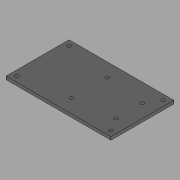
# Autodesk Inventor part: rfid_cover
Saved by Autodesk Inventor 2019 (Build 230136000, 136)
## iProperties
Part Number: rfid_cover
Material: Generic
Document SubType Name: Modeling
Designer: Javi
Appearance: Default
Author: Javi
Autodesk Inventor part; units mm, degrees
ref_plane "YZ Plane" through (0, 0, 0) normal (1, 0, 0) x (0, 1, 0)
ref_plane "XZ Plane" through (0, 0, 0) normal (0, 1, 0) x (-1, 0, 0)
ref_plane "XY Plane" through (0, 0, 0) normal (0, 0, 1) x (1, 0, 0)
sketch "Sketch1" plane through (0, 0, 0) normal (0, 1, 0) x (-1, 0, 0)
  line L0 (0, -60) -> (-100, -60)
  line L1 (-100, -60) -> (-100, 0)
  line L2 (-100, 0) -> (0, 0)
  line L3 (0, 0) -> (0, -60)
  dimension "d0" = 100
  dimension "d1" = 60
  constraints: 8 end point, 2 parallel, 1 coincident, 1 horizontal, 1 perpendicular
  measures "d0" distance of L0.start L0.end
  measures "d1" distance of L0.end L1.end
extrude "Extrusion1" add sketch "Sketch1" along normal blind 3
sketch "Sketch2" plane through (0, 3, 0) normal (0, 1, 0) x (1, 0, 0)
  circle A0 centre (5, 55) radius 1.75
  line L0 (100, 60) -> (0, 60) projected
  line L1 (0, 60) -> (0, 0) projected
  circle A1 centre (95, 55) radius 1.75
  circle A2 centre (5, 5) radius 1.75
  circle A3 centre (95, 5) radius 1.75
  circle A4 centre (87.5, 42.5) radius 1.75
  circle A5 centre (87.5, 17.5) radius 1.75
  line L2 (100, 0) -> (100, 60) projected
  circle A6 centre (49.5, 47) radius 1.75
  circle A7 centre (49.5, 13) radius 1.75
  dimension "d4" = 3.5
  dimension "d5" = 5
  dimension "d6" = 5
  dimension "d9" = 90
  dimension "d12" = 50
  dimension "d15" = 3.5
  dimension "d16" = 3.5
  dimension "d17" = 25
  dimension "d18" = 0
  dimension "d19" = 12.5
  dimension "d20" = 3.5
  dimension "d21" = 3.5
  dimension "d22" = 34
  dimension "d23" = 0
  dimension "d24" = 38
  dimension "d25" = 17.5
  dimension "d26" = 13
  constraints: 8 centre point, 1 horizontal, 1 vertical, 6 other
  measures "d4" diameter of A0
  measures "d5" distance from line of L0 A0.centre
  measures "d6" distance from line of L1 A0.centre
  measures "d9" distance of A0.centre A1.centre
  measures "d12" distance of A0.centre A2.centre
  measures "d15" diameter of A4
  measures "d16" diameter of A5
  measures "d17" distance of A4.centre A5.centre
  measures "d18" horizontal distance of A5.centre A4.centre
  measures "d19" distance from line of L2 A4.centre
  measures "d20" diameter of A6
  measures "d21" diameter of A7
  measures "d22" distance of A7.centre A6.centre
  measures "d23" horizontal distance of A7.centre A6.centre
  measures "d24" horizontal distance of A4.centre A6.centre
  measures "d25" distance from line of L0 A4.centre
  measures "d26" distance from line of L0 A6.centre
extrude "Extrusion2" cut sketch "Sketch2" against normal through all
body "Solid1"
